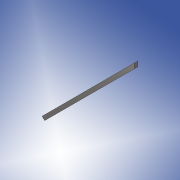
# Autodesk Inventor part: C004
Saved by Autodesk Inventor 2017 (Build 210142000, 142)
## iProperties
Created: 2017-06-13
Part Number: C004
Material: Steel, Carbon
Document SubType Name: Modeling
Designer: zallen
Density: 7.85 g/cm^3
Appearance: Semi-Polished
Author: zallen
Autodesk Inventor part; units mm, degrees
ref_plane "YZ Plane" through (0, 0, 0) normal (1, 0, 0) x (0, 1, 0)
ref_plane "XZ Plane" through (0, 0, 0) normal (0, 1, 0) x (-1, 0, 0)
ref_plane "XY Plane" through (0, 0, 0) normal (0, 0, 1) x (1, 0, 0)
sketch "Sketch2" plane through (0, 0, 0) normal (0, 0, 1) x (1, 0, 0)
  line L0 (0, 0) -> (377.5, 0) construction
  line L1 (377.5, 0) -> (377.5, 377.5) construction
  line L2 (0, 0) -> (377.5, 377.5) construction
  line L3 (-5.3033, 5.3033) -> (5.3033, -5.3033)
  line L4 (377.5, 388.1066) -> (377.5, 366.8934)
  line L5 (-5.3033, 5.3033) -> (377.5, 388.1066)
  line L6 (5.3033, -5.3033) -> (377.5, 366.8934)
  dimension "d4" = 377.5
  dimension "d5" = 377.5
  dimension "d6" = 15
  dimension "d7" = 90
  dimension "d13" = 45
  constraints: 14 end point, 2 midpoint, 1 horizontal, 1 perpendicular, 1 point on line
  measures "d4" distance of L0.start L0.end
  measures "d5" distance of L1.end L0.end
  measures "d6" distance of L3.start L3.end
  measures "d7" angle of L2 L3
  measures "d13" angle of L0 L6
extrude "Extrusion1" add sketch "Sketch2" along normal blind 15
body "Solid1"
